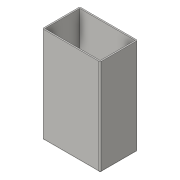
# Autodesk Inventor part: Case
Saved by Autodesk Inventor 2016 SP2 (Build 200236200, 236)
## iProperties
Created: 2017-04-16
Part Number: Case
Material: Generic
Document SubType Name: Modeling
Designer: Karl
Density: 1 g/cm^3
Appearance: Default
Author: Karl
Autodesk Inventor part; units mm, degrees
ref_plane "YZ Plane" through (0, 0, 0) normal (1, 0, 0) x (0, 1, 0)
ref_plane "XZ Plane" through (0, 0, 0) normal (0, 1, 0) x (-1, 0, 0)
ref_plane "XY Plane" through (0, 0, 0) normal (0, 0, 1) x (1, 0, 0)
sketch "Sketch2" plane through (0, 0, 0) normal (0, 1, 0) x (-1, 0, 0)
  line L0 (-21.25, -13.75) -> (21.25, -13.75)
  line L1 (21.25, -13.75) -> (21.25, 13.75)
  line L2 (21.25, 13.75) -> (-21.25, 13.75)
  line L3 (-21.25, 13.75) -> (-21.25, -13.75)
  line L4 (-21.25, -13.75) -> (21.25, 13.75) construction
  line L5 (21.25, -13.75) -> (-21.25, 13.75) construction
  point P0 (0, 0)
  dimension "d2" = 42.5
  dimension "d3" = 27.5
  constraints: 12 end point, 2 midpoint, 2 parallel, 1 horizontal, 1 perpendicular
  measures "d2" distance of L2.end L1.end
  measures "d3" distance of L2.end L0.start
extrude "Extrusion1" add sketch "Sketch2" against normal blind 2
sketch "Sketch3" plane through (0, 0, 0) normal (0, 1, 0) x (1, 0, 0)
  line L0 (21.25, -13.75) -> (-21.25, -13.75) projected
  line L1 (-21.25, 13.75) -> (21.25, 13.75) projected
  line L2 (-21.25, -13.75) -> (21.25, -13.75)
  line L3 (21.25, -13.75) -> (21.25, 13.75)
  line L4 (21.25, 13.75) -> (-21.25, 13.75)
  line L5 (-21.25, 13.75) -> (-21.25, -13.75)
  line L6 (-20.25, -12.75) -> (20.25, -12.75) projected
  line L7 (-20.25, 12.75) -> (-20.25, -12.75) projected
  line L8 (20.25, 12.75) -> (-20.25, 12.75) projected
  line L9 (20.25, -12.75) -> (20.25, 12.75) projected
  line L10 (-20.25, -12.75) -> (20.25, -12.75)
  line L11 (20.25, -12.75) -> (20.25, 12.75)
  line L12 (20.25, 12.75) -> (-20.25, 12.75)
  line L13 (-20.25, 12.75) -> (-20.25, -12.75)
  point P0 (0, 0)
  constraints: 16 end point, 4 parallel, 2 horizontal, 2 perpendicular
extrude "Extrusion2" add sketch "Sketch3" along normal blind 60.5
fillet "Fillet1" radius 1 8 edges at (21.25, 29.25, 13.75) (21.25, 29.25, -13.75) (-21.25, 29.25, 13.75) (-21.25, 29.25, -13.75) (0, -2, -13.75) (21.25, -2, 0) (0, -2, 13.75) (-21.25, -2, 0)
sketch "Sketch4" plane through (0, 60.5, 0) normal (0, 1, 0) x (1, 0, 0)
  arc A0 (-20.25, 13.75) -> (-21.25, 12.75) centre (-20.25, 12.75) ccw projected
  line L0 (-21.25, 12.75) -> (-21.25, -12.75) projected
  arc A1 (-21.25, -12.75) -> (-20.25, -13.75) centre (-20.25, -12.75) ccw projected
  line L1 (-20.25, -13.75) -> (20.25, -13.75) projected
  arc A2 (20.25, -13.75) -> (21.25, -12.75) centre (20.25, -12.75) ccw projected
  line L2 (21.25, -12.75) -> (21.25, 12.75) projected
  arc A3 (21.25, 12.75) -> (20.25, 13.75) centre (20.25, 12.75) ccw projected
  line L3 (20.25, 13.75) -> (-20.25, 13.75) projected
  line L4 (-20.25, -12.75) -> (-20.25, 12.75) projected
  line L5 (-20.25, 12.75) -> (20.25, 12.75) projected
  line L6 (20.25, 12.75) -> (20.25, -12.75) projected
  line L7 (20.25, -12.75) -> (-20.25, -12.75) projected
  point P0 (0, 0)
extrude "Extrusion3" add sketch "Sketch4" along normal blind 8
body "Solid1"
